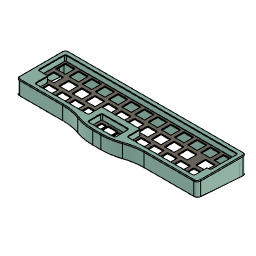
threeu v1 (Autodesk Fusion 360 design; units mm, degrees)
Autodesk Fusion 360 part; units mm, degrees
sketch "plate-2023-07-07T18_42_50.088Z" plane through (0, 0, 0) normal (0, 0, 1) x (1, 0, 0) in component "threeu"
  line L0 (40.625, -3.025) -> (40.625, -16.025)
  line L1 (3.025, -2.525) -> (16.025, -2.525)
  arc A0 (21.575, -16.025) -> (22.075, -16.525) centre (22.075, -16.025) ccw
  arc A1 (59.675, -16.025) -> (60.175, -16.525) centre (60.175, -16.025) ccw
  arc A2 (79.225, -2.525) -> (78.725, -3.025) centre (79.225, -3.025) ccw
  line L2 (98.275, -16.525) -> (111.275, -16.525)
  arc A3 (35.575, -3.025) -> (35.075, -2.525) centre (35.075, -3.025) ccw
  arc A4 (54.125, -16.525) -> (54.625, -16.025) centre (54.125, -16.025) ccw
  line L3 (97.775, -3.025) -> (97.775, -16.025)
  arc A5 (111.775, -3.025) -> (111.275, -2.525) centre (111.275, -3.025) ccw
  arc A6 (111.275, -16.525) -> (111.775, -16.025) centre (111.275, -16.025) ccw
  arc A7 (117.325, -2.525) -> (116.825, -3.025) centre (117.325, -3.025) ccw
  line L4 (136.375, -16.525) -> (149.375, -16.525)
  line L5 (35.575, -3.025) -> (35.575, -16.025)
  line L6 (3.025, -16.525) -> (16.025, -16.525)
  arc A8 (73.175, -16.525) -> (73.675, -16.025) centre (73.175, -16.025) ccw
  line L7 (92.725, -3.025) -> (92.725, -16.025)
  line L8 (135.875, -3.025) -> (135.875, -16.025)
  line L9 (149.875, -3.025) -> (149.875, -16.025)
  line L10 (60.175, -2.525) -> (73.175, -2.525)
  arc A9 (136.375, -2.525) -> (135.875, -3.025) centre (136.375, -3.025) ccw
  line L11 (73.675, -3.025) -> (73.675, -16.025)
  arc A10 (92.225, -16.525) -> (92.725, -16.025) centre (92.225, -16.025) ccw
  arc A11 (16.525, -3.025) -> (16.025, -2.525) centre (16.025, -3.025) ccw
  line L12 (79.225, -2.525) -> (92.225, -2.525)
  line L13 (79.225, -16.525) -> (92.225, -16.525)
  line L14 (22.075, -16.525) -> (35.075, -16.525)
  arc A12 (92.725, -3.025) -> (92.225, -2.525) centre (92.225, -3.025) ccw
  line L15 (111.775, -3.025) -> (111.775, -16.025)
  arc A13 (22.075, -2.525) -> (21.575, -3.025) centre (22.075, -3.025) ccw
  line L16 (21.575, -3.025) -> (21.575, -16.025)
  line L17 (98.275, -2.525) -> (111.275, -2.525)
  arc A14 (73.675, -3.025) -> (73.175, -2.525) centre (73.175, -3.025) ccw
  line L18 (136.375, -2.525) -> (149.375, -2.525)
  arc A15 (3.025, -2.525) -> (2.525, -3.025) centre (3.025, -3.025) ccw
  line L19 (2.525, -3.025) -> (2.525, -16.025)
  line L20 (54.625, -3.025) -> (54.625, -16.025)
  arc A16 (40.625, -16.025) -> (41.125, -16.525) centre (41.125, -16.025) ccw
  line L21 (41.125, -2.525) -> (54.125, -2.525)
  arc A17 (35.075, -16.525) -> (35.575, -16.025) centre (35.075, -16.025) ccw
  arc A18 (16.025, -16.525) -> (16.525, -16.025) centre (16.025, -16.025) ccw
  arc A19 (116.825, -16.025) -> (117.325, -16.525) centre (117.325, -16.025) ccw
  line L22 (174.475, -16.525) -> (187.475, -16.525)
  line L23 (16.525, -3.025) -> (16.525, -16.025)
  arc A20 (60.175, -2.525) -> (59.675, -3.025) centre (60.175, -3.025) ccw
  arc A21 (212.575, -2.525) -> (212.075, -3.025) centre (212.575, -3.025) ccw
  line L24 (130.825, -3.025) -> (130.825, -16.025)
  line L25 (117.325, -2.525) -> (130.325, -2.525)
  line L26 (117.325, -16.525) -> (130.325, -16.525)
  line L27 (22.075, -2.525) -> (35.075, -2.525)
  line L28 (59.675, -3.025) -> (59.675, -16.025)
  arc A22 (149.375, -16.525) -> (149.875, -16.025) centre (149.375, -16.025) ccw
  line L29 (193.025, -3.025) -> (193.025, -16.025)
  arc A23 (245.125, -3.025) -> (244.625, -2.525) centre (244.625, -3.025) ccw
  arc A24 (78.725, -16.025) -> (79.225, -16.525) centre (79.225, -16.025) ccw
  arc A25 (98.275, -2.525) -> (97.775, -3.025) centre (98.275, -3.025) ccw
  arc A26 (41.125, -2.525) -> (40.625, -3.025) centre (41.125, -3.025) ccw
  line L30 (116.825, -3.025) -> (116.825, -16.025)
  arc A27 (231.125, -16.025) -> (231.625, -16.525) centre (231.625, -16.025) ccw
  arc A28 (18.9062, -22.075) -> (18.4062, -21.575) centre (18.4062, -22.075) ccw
  arc A29 (130.825, -3.025) -> (130.325, -2.525) centre (130.325, -3.025) ccw
  arc A30 (130.325, -16.525) -> (130.825, -16.025) centre (130.325, -16.025) ccw
  arc A31 (18.4062, -35.575) -> (18.9062, -35.075) centre (18.4062, -35.075) ccw
  line L31 (45.8875, -21.575) -> (58.8875, -21.575)
  line L32 (154.925, -3.025) -> (154.925, -16.025)
  arc A32 (97.775, -16.025) -> (98.275, -16.525) centre (98.275, -16.025) ccw
  arc A33 (193.525, -2.525) -> (193.025, -3.025) centre (193.525, -3.025) ccw
  arc A34 (40.3375, -22.075) -> (39.8375, -21.575) centre (39.8375, -22.075) ccw
  line L33 (212.075, -3.025) -> (212.075, -16.025)
  line L34 (174.475, -2.525) -> (187.475, -2.525)
  arc A35 (207.025, -3.025) -> (206.525, -2.525) centre (206.525, -3.025) ccw
  line L35 (41.125, -16.525) -> (54.125, -16.525)
  arc A36 (231.625, -2.525) -> (231.125, -3.025) centre (231.625, -3.025) ccw
  arc A37 (54.625, -3.025) -> (54.125, -2.525) centre (54.125, -3.025) ccw
  line L36 (78.725, -3.025) -> (78.725, -16.025)
  line L37 (231.125, -3.025) -> (231.125, -16.025)
  arc A38 (149.875, -3.025) -> (149.375, -2.525) centre (149.375, -3.025) ccw
  arc A39 (135.875, -16.025) -> (136.375, -16.525) centre (136.375, -16.025) ccw
  arc A40 (155.425, -2.525) -> (154.925, -3.025) centre (155.425, -3.025) ccw
  line L38 (26.8375, -21.575) -> (39.8375, -21.575)
  line L39 (26.3375, -22.075) -> (26.3375, -35.075)
  line L40 (18.9063, -22.075) -> (18.9063, -35.075)
  line L41 (60.175, -16.525) -> (73.175, -16.525)
  line L42 (155.425, -16.525) -> (168.425, -16.525)
  arc A41 (2.525, -16.025) -> (3.025, -16.525) centre (3.025, -16.025) ccw
  arc A42 (212.075, -16.025) -> (212.575, -16.525) centre (212.575, -16.025) ccw
  arc A43 (5.4062, -21.575) -> (4.9063, -22.075) centre (5.4062, -22.075) ccw
  line L43 (45.8875, -35.575) -> (58.8875, -35.575)
  line L44 (5.4062, -35.575) -> (18.4063, -35.575)
  line L45 (212.575, -2.525) -> (225.575, -2.525)
  line L46 (59.3875, -22.075) -> (59.3875, -35.075)
  arc A44 (193.025, -16.025) -> (193.525, -16.525) centre (193.525, -16.025) ccw
  line L47 (45.3875, -22.075) -> (45.3875, -35.075)
  line L48 (193.525, -2.525) -> (206.525, -2.525)
  arc A45 (45.8875, -21.575) -> (45.3875, -22.075) centre (45.8875, -22.075) ccw
  line L49 (212.575, -16.525) -> (225.575, -16.525)
  line L50 (187.975, -3.025) -> (187.975, -16.025)
  line L51 (173.975, -3.025) -> (173.975, -16.025)
  arc A46 (187.475, -16.525) -> (187.975, -16.025) centre (187.475, -16.025) ccw
  line L52 (207.025, -3.025) -> (207.025, -16.025)
  arc A47 (168.425, -16.525) -> (168.925, -16.025) centre (168.425, -16.025) ccw
  line L53 (245.125, -3.025) -> (245.125, -16.025)
  line L54 (226.075, -3.025) -> (226.075, -16.025)
  arc A48 (225.575, -16.525) -> (226.075, -16.025) centre (225.575, -16.025) ccw
  line L55 (26.8375, -35.575) -> (39.8375, -35.575)
  line L56 (168.925, -3.025) -> (168.925, -16.025)
  line L57 (231.625, -2.525) -> (244.625, -2.525)
  line L58 (4.9062, -22.075) -> (4.9062, -35.075)
  line L59 (193.525, -16.525) -> (206.525, -16.525)
  arc A49 (174.475, -2.525) -> (173.975, -3.025) centre (174.475, -3.025) ccw
  arc A50 (226.075, -3.025) -> (225.575, -2.525) centre (225.575, -3.025) ccw
  arc A51 (4.9062, -35.075) -> (5.4062, -35.575) centre (5.4062, -35.075) ccw
  line L60 (40.3375, -22.075) -> (40.3375, -35.075)
  line L61 (5.4062, -21.575) -> (18.4063, -21.575)
  arc A52 (168.925, -3.025) -> (168.425, -2.525) centre (168.425, -3.025) ccw
  line L62 (231.625, -16.525) -> (244.625, -16.525)
  line L63 (155.425, -2.525) -> (168.425, -2.525)
  arc A53 (26.3375, -35.075) -> (26.8375, -35.575) centre (26.8375, -35.075) ccw
  arc A54 (39.8375, -35.575) -> (40.3375, -35.075) centre (39.8375, -35.075) ccw
  arc A55 (187.975, -3.025) -> (187.475, -2.525) centre (187.475, -3.025) ccw
  arc A56 (244.625, -16.525) -> (245.125, -16.025) centre (244.625, -16.025) ccw
  arc A57 (26.8375, -21.575) -> (26.3375, -22.075) centre (26.8375, -22.075) ccw
  arc A58 (160.1875, -21.575) -> (159.6875, -22.075) centre (160.1875, -22.075) ccw
  arc A59 (173.975, -16.025) -> (174.475, -16.525) centre (174.475, -16.025) ccw
  arc A60 (206.525, -16.525) -> (207.025, -16.025) centre (206.525, -16.025) ccw
  line L64 (103.0375, -21.575) -> (116.0375, -21.575)
  line L65 (192.7375, -22.075) -> (192.7375, -35.075)
  line L66 (160.1875, -21.575) -> (173.1875, -21.575)
  arc A61 (178.7375, -35.075) -> (179.2375, -35.575) centre (179.2375, -35.075) ccw
  arc A62 (154.925, -16.025) -> (155.425, -16.525) centre (155.425, -16.025) ccw
  arc A63 (140.6375, -35.075) -> (141.1375, -35.575) centre (141.1375, -35.075) ccw
  arc A64 (135.5875, -22.075) -> (135.0875, -21.575) centre (135.0875, -22.075) ccw
  arc A65 (141.1375, -21.575) -> (140.6375, -22.075) centre (141.1375, -22.075) ccw
  line L67 (141.1375, -21.575) -> (154.1375, -21.575)
  arc A66 (192.2375, -35.575) -> (192.7375, -35.075) centre (192.2375, -35.075) ccw
  line L68 (64.9375, -35.575) -> (77.9375, -35.575)
  arc A67 (159.6875, -35.075) -> (160.1875, -35.575) centre (160.1875, -35.075) ccw
  line L69 (159.6875, -22.075) -> (159.6875, -35.075)
  line L70 (83.9875, -35.575) -> (96.9875, -35.575)
  line L71 (64.9375, -21.575) -> (77.9375, -21.575)
  arc A68 (192.7375, -22.075) -> (192.2375, -21.575) centre (192.2375, -22.075) ccw
  line L72 (198.2875, -21.575) -> (211.2875, -21.575)
  line L73 (97.4875, -22.075) -> (97.4875, -35.075)
  arc A69 (59.3875, -22.075) -> (58.8875, -21.575) centre (58.8875, -22.075) ccw
  arc A70 (58.8875, -35.575) -> (59.3875, -35.075) centre (58.8875, -35.075) ccw
  line L74 (179.2375, -35.575) -> (192.2375, -35.575)
  arc A71 (154.6375, -22.075) -> (154.1375, -21.575) centre (154.1375, -22.075) ccw
  line L75 (179.2375, -21.575) -> (192.2375, -21.575)
  line L76 (197.7875, -22.075) -> (197.7875, -35.075)
  line L77 (140.6375, -22.075) -> (140.6375, -35.075)
  line L78 (198.2875, -35.575) -> (211.2875, -35.575)
  line L79 (135.5875, -22.075) -> (135.5875, -35.075)
  line L80 (102.5375, -22.075) -> (102.5375, -35.075)
  arc A72 (173.6875, -22.075) -> (173.1875, -21.575) centre (173.1875, -22.075) ccw
  line L81 (154.6375, -22.075) -> (154.6375, -35.075)
  arc A73 (64.9375, -21.575) -> (64.4375, -22.075) centre (64.9375, -22.075) ccw
  line L82 (160.1875, -35.575) -> (173.1875, -35.575)
  arc A74 (179.2375, -21.575) -> (178.7375, -22.075) centre (179.2375, -22.075) ccw
  line L83 (211.7875, -22.075) -> (211.7875, -35.075)
  arc A75 (122.0875, -21.575) -> (121.5875, -22.075) centre (122.0875, -22.075) ccw
  arc A76 (97.4875, -22.075) -> (96.9875, -21.575) centre (96.9875, -22.075) ccw
  line L84 (122.0875, -35.575) -> (135.0875, -35.575)
  line L85 (178.7375, -22.075) -> (178.7375, -35.075)
  arc A77 (103.0375, -21.575) -> (102.5375, -22.075) centre (103.0375, -22.075) ccw
  line L86 (83.9875, -21.575) -> (96.9875, -21.575)
  line L87 (116.5375, -22.075) -> (116.5375, -35.075)
  line L88 (83.4875, -22.075) -> (83.4875, -35.075)
  line L89 (141.1375, -35.575) -> (154.1375, -35.575)
  arc A78 (96.9875, -35.575) -> (97.4875, -35.075) centre (96.9875, -35.075) ccw
  line L90 (17.3125, -40.625) -> (30.3125, -40.625)
  arc A79 (223.9813, -35.075) -> (224.4813, -35.575) centre (224.4813, -35.075) ccw
  line L91 (103.0375, -35.575) -> (116.0375, -35.575)
  arc A80 (116.5375, -22.075) -> (116.0375, -21.575) centre (116.0375, -22.075) ccw
  arc A81 (77.9375, -35.575) -> (78.4375, -35.075) centre (77.9375, -35.075) ccw
  line L92 (122.0875, -21.575) -> (135.0875, -21.575)
  arc A82 (78.4375, -22.075) -> (77.9375, -21.575) centre (77.9375, -22.075) ccw
  arc A83 (188.7625, -40.625) -> (188.2625, -41.125) centre (188.7625, -41.125) ccw
  arc A84 (45.3875, -35.075) -> (45.8875, -35.575) centre (45.8875, -35.075) ccw
  arc A85 (121.5875, -35.075) -> (122.0875, -35.575) centre (122.0875, -35.075) ccw
  line L93 (183.2125, -41.125) -> (183.2125, -54.125)
  arc A86 (154.1375, -35.575) -> (154.6375, -35.075) centre (154.1375, -35.075) ccw
  line L94 (173.6875, -22.075) -> (173.6875, -35.075)
  arc A87 (87.9625, -41.125) -> (87.4625, -40.625) centre (87.4625, -41.125) ccw
  arc A88 (198.2875, -21.575) -> (197.7875, -22.075) centre (198.2875, -22.075) ccw
  line L95 (121.5875, -22.075) -> (121.5875, -35.075)
  arc A89 (83.4875, -35.075) -> (83.9875, -35.575) centre (83.9875, -35.075) ccw
  arc A90 (68.9125, -41.125) -> (68.4125, -40.625) centre (68.4125, -41.125) ccw
  arc A91 (211.7875, -22.075) -> (211.2875, -21.575) centre (211.2875, -22.075) ccw
  arc A92 (164.1625, -41.125) -> (163.6625, -40.625) centre (163.6625, -41.125) ccw
  line L96 (150.6625, -40.625) -> (163.6625, -40.625)
  arc A93 (237.9813, -22.075) -> (237.4813, -21.575) centre (237.4813, -22.075) ccw
  line L97 (78.4375, -22.075) -> (78.4375, -35.075)
  line L98 (64.4375, -22.075) -> (64.4375, -35.075)
  line L99 (202.2625, -41.125) -> (202.2625, -54.125)
  arc A94 (83.9875, -21.575) -> (83.4875, -22.075) centre (83.9875, -22.075) ccw
  arc A95 (173.1875, -35.575) -> (173.6875, -35.075) centre (173.1875, -35.075) ccw
  arc A96 (116.0375, -35.575) -> (116.5375, -35.075) centre (116.0375, -35.075) ccw
  arc A97 (135.0875, -35.575) -> (135.5875, -35.075) centre (135.0875, -35.075) ccw
  arc A98 (87.4625, -54.625) -> (87.9625, -54.125) centre (87.4625, -54.125) ccw
  arc A99 (64.4375, -35.075) -> (64.9375, -35.575) centre (64.9375, -35.075) ccw
  arc A100 (102.5375, -35.075) -> (103.0375, -35.575) centre (103.0375, -35.075) ccw
  line L100 (49.8625, -41.125) -> (49.8625, -54.125)
  arc A101 (16.8125, -54.125) -> (17.3125, -54.625) centre (17.3125, -54.125) ccw
  line L101 (36.3625, -40.625) -> (49.3625, -40.625)
  arc A102 (49.3625, -54.625) -> (49.8625, -54.125) centre (49.3625, -54.125) ccw
  line L102 (74.4625, -54.625) -> (87.4625, -54.625)
  line L103 (223.9812, -22.075) -> (223.9812, -35.075)
  line L104 (16.8125, -41.125) -> (16.8125, -54.125)
  arc A103 (17.3125, -40.625) -> (16.8125, -41.125) centre (17.3125, -41.125) ccw
  arc A104 (224.4813, -21.575) -> (223.9813, -22.075) centre (224.4813, -22.075) ccw
  arc A105 (36.3625, -40.625) -> (35.8625, -41.125) centre (36.3625, -41.125) ccw
  line L105 (54.9125, -41.125) -> (54.9125, -54.125)
  arc A106 (55.4125, -40.625) -> (54.9125, -41.125) centre (55.4125, -41.125) ccw
  line L106 (30.8125, -41.125) -> (30.8125, -54.125)
  arc A107 (73.9625, -54.125) -> (74.4625, -54.625) centre (74.4625, -54.125) ccw
  arc A108 (68.4125, -54.625) -> (68.9125, -54.125) centre (68.4125, -54.125) ccw
  line L107 (55.4125, -40.625) -> (68.4125, -40.625)
  arc A109 (197.7875, -35.075) -> (198.2875, -35.575) centre (198.2875, -35.075) ccw
  line L108 (36.3625, -54.625) -> (49.3625, -54.625)
  line L109 (164.1625, -41.125) -> (164.1625, -54.125)
  arc A110 (150.6625, -40.625) -> (150.1625, -41.125) centre (150.6625, -41.125) ccw
  arc A111 (30.8125, -41.125) -> (30.3125, -40.625) centre (30.3125, -41.125) ccw
  line L110 (237.9813, -22.075) -> (237.9812, -35.075)
  arc A112 (237.4813, -35.575) -> (237.9813, -35.075) centre (237.4813, -35.075) ccw
  line L111 (35.8625, -41.125) -> (35.8625, -54.125)
  line L112 (150.6625, -54.625) -> (163.6625, -54.625)
  line L113 (74.4625, -40.625) -> (87.4625, -40.625)
  line L114 (55.4125, -54.625) -> (68.4125, -54.625)
  line L115 (169.7125, -40.625) -> (182.7125, -40.625)
  arc A113 (169.7125, -40.625) -> (169.2125, -41.125) centre (169.7125, -41.125) ccw
  arc A114 (169.2125, -54.125) -> (169.7125, -54.625) centre (169.7125, -54.125) ccw
  arc A115 (182.7125, -54.625) -> (183.2125, -54.125) centre (182.7125, -54.125) ccw
  arc A116 (211.2875, -35.575) -> (211.7875, -35.075) centre (211.2875, -35.075) ccw
  arc A117 (30.3125, -54.625) -> (30.8125, -54.125) centre (30.3125, -54.125) ccw
  line L116 (68.9125, -41.125) -> (68.9125, -54.125)
  line L117 (73.9625, -41.125) -> (73.9625, -54.125)
  arc A118 (150.1625, -54.125) -> (150.6625, -54.625) centre (150.6625, -54.125) ccw
  line L118 (150.1625, -41.125) -> (150.1625, -54.125)
  line L119 (169.2125, -41.125) -> (169.2125, -54.125)
  arc A119 (183.2125, -41.125) -> (182.7125, -40.625) centre (182.7125, -41.125) ccw
  line L120 (224.4813, -35.575) -> (237.4813, -35.575)
  line L121 (87.9625, -41.125) -> (87.9625, -54.125)
  line L122 (17.3125, -54.625) -> (30.3125, -54.625)
  arc A120 (54.9125, -54.125) -> (55.4125, -54.625) centre (55.4125, -54.125) ccw
  arc A121 (163.6625, -54.625) -> (164.1625, -54.125) centre (163.6625, -54.125) ccw
  arc A122 (35.8625, -54.125) -> (36.3625, -54.625) centre (36.3625, -54.125) ccw
  arc A123 (49.8625, -41.125) -> (49.3625, -40.625) centre (49.3625, -41.125) ccw
  line L123 (188.2625, -41.125) -> (188.2625, -54.125)
  arc A124 (74.4625, -40.625) -> (73.9625, -41.125) centre (74.4625, -41.125) ccw
  line L124 (224.4813, -21.575) -> (237.4813, -21.575)
  line L125 (169.7125, -54.625) -> (182.7125, -54.625)
  line L126 (188.7625, -40.625) -> (201.7625, -40.625)
  line L127 (188.7625, -54.625) -> (201.7625, -54.625)
  line L128 (112.0625, -50.65) -> (112.0625, -63.65)
  line L129 (128.0005, -51.15) -> (134.0005, -51.15)
  arc A125 (110.6245, -51.65) -> (110.1245, -51.15) centre (110.1245, -51.65) ccw
  arc A126 (134.5005, -51.65) -> (134.0005, -51.15) centre (134.0005, -51.65) ccw
  arc A127 (221.3125, -41.125) -> (220.8125, -40.625) centre (220.8125, -41.125) ccw
  line L130 (100.0125, -66.675) -> (138.1125, -66.675)
  arc A128 (112.0625, -63.65) -> (112.5625, -64.15) centre (112.5625, -63.65) ccw
  arc A129 (201.7625, -54.625) -> (202.2625, -54.125) centre (201.7625, -54.125) ccw
  line L131 (134.5005, -51.65) -> (134.5005, -65.65)
  arc A130 (239.8625, -54.625) -> (240.3625, -54.125) centre (239.8625, -54.125) ccw
  line L132 (127.5005, -51.65) -> (127.5005, -65.65)
  line L133 (0, 0) -> (247.65, 0)
  arc A131 (127.5005, -65.65) -> (128.0005, -66.15) centre (128.0005, -65.65) ccw
  line L134 (126.0625, -50.65) -> (126.0625, -63.65)
  line L135 (226.8625, -40.625) -> (239.8625, -40.625)
  arc A132 (226.8625, -40.625) -> (226.3625, -41.125) centre (226.8625, -41.125) ccw
  arc A133 (110.1245, -66.15) -> (110.6245, -65.65) centre (110.1245, -65.65) ccw
  line L136 (240.3625, -41.125) -> (240.3625, -54.125)
  arc A134 (226.3625, -54.125) -> (226.8625, -54.625) centre (226.8625, -54.125) ccw
  line L137 (221.3125, -41.125) -> (221.3125, -54.125)
  arc A135 (125.5625, -64.15) -> (126.0625, -63.65) centre (125.5625, -63.65) ccw
  line L138 (128.0005, -66.15) -> (134.0005, -66.15)
  arc A136 (220.8125, -54.625) -> (221.3125, -54.125) centre (220.8125, -54.125) ccw
  arc A137 (126.0625, -50.65) -> (125.5625, -50.15) centre (125.5625, -50.65) ccw
  line L139 (104.1245, -66.15) -> (110.1245, -66.15)
  arc A138 (112.5625, -50.15) -> (112.0625, -50.65) centre (112.5625, -50.65) ccw
  line L140 (110.6245, -51.65) -> (110.6245, -65.65)
  arc A139 (103.6245, -65.65) -> (104.1245, -66.15) centre (104.1245, -65.65) ccw
  arc A140 (202.2625, -41.125) -> (201.7625, -40.625) centre (201.7625, -41.125) ccw
  line L141 (226.8625, -54.625) -> (239.8625, -54.625)
  line L142 (207.8125, -54.625) -> (220.8125, -54.625)
  arc A141 (207.8125, -40.625) -> (207.3125, -41.125) centre (207.8125, -41.125) ccw
  line L143 (226.3625, -41.125) -> (226.3625, -54.125)
  arc A142 (207.3125, -54.125) -> (207.8125, -54.625) centre (207.8125, -54.125) ccw
  arc A143 (188.2625, -54.125) -> (188.7625, -54.625) centre (188.7625, -54.125) ccw
  line L144 (207.8125, -40.625) -> (220.8125, -40.625)
  line L145 (112.5625, -50.15) -> (125.5625, -50.15)
  line L146 (104.1245, -51.15) -> (110.1245, -51.15)
  arc A144 (134.0005, -66.15) -> (134.5005, -65.65) centre (134.0005, -65.65) ccw
  line L147 (0, -38.1) -> (0, 0)
  arc A145 (128.0005, -51.15) -> (127.5005, -51.65) centre (128.0005, -51.65) ccw
  line L148 (207.3125, -41.125) -> (207.3125, -54.125)
  line L149 (103.6245, -51.65) -> (103.6245, -65.65)
  arc A146 (104.1245, -51.15) -> (103.6245, -51.65) centre (104.1245, -51.65) ccw
  arc A147 (240.3625, -41.125) -> (239.8625, -40.625) centre (239.8625, -41.125) ccw
  line L150 (112.5625, -64.15) -> (125.5625, -64.15)
  line L151 (247.65, -38.1) -> (247.65, 0)
  line L152 (33.3375, -57.15) -> (14.2875, -57.15)
  line L153 (14.2875, -57.15) -> (14.2875, -38.1)
  line L154 (14.2875, -38.1) -> (33.3375, -57.15) construction
  line L155 (33.3375, -38.1) -> (14.2875, -57.15) construction
  line L156 (242.8875, -57.15) -> (223.8375, -57.15)
  line L157 (242.8875, -38.1) -> (242.8875, -57.15)
  line L158 (242.8875, -57.15) -> (223.8375, -38.1) construction
  line L159 (223.8375, -57.15) -> (242.8875, -38.1) construction
  line L160 (242.8875, -38.1) -> (247.65, -38.1)
  line L161 (138.1125, -66.675) -> (100.0125, -66.675)
  line L162 (100.0125, -66.675) -> (100.0125, -47.625)
  line L163 (100.0125, -47.625) -> (138.1125, -47.625)
  line L164 (138.1125, -47.625) -> (138.1125, -66.675)
  line L165 (138.1125, -66.675) -> (100.0125, -47.625) construction
  line L166 (100.0125, -66.675) -> (138.1125, -47.625) construction
  line L167 (90.4875, -57.15) -> (71.4375, -57.15)
  line L168 (90.4875, -38.1) -> (90.4875, -57.15)
  line L169 (90.4875, -57.15) -> (71.4375, -38.1) construction
  line L170 (71.4375, -57.15) -> (90.4875, -38.1) construction
  line L171 (147.6375, -57.15) -> (166.6875, -57.15)
  line L172 (147.6375, -38.1) -> (147.6375, -57.15)
  line L173 (147.6375, -57.15) -> (166.6875, -38.1) construction
  line L174 (166.6875, -57.15) -> (147.6375, -38.1) construction
  line L175 (147.6375, -38.1) -> (90.4875, -38.1)
  line L176 (71.4375, -57.15) -> (33.3375, -57.15)
  line L177 (14.2875, -38.1) -> (0, -38.1)
  line L178 (166.6875, -57.15) -> (223.8375, -57.15)
  line L179 (138.1125, -66.675) -> (147.6375, -57.15)
  line L180 (100.0125, -66.675) -> (90.4875, -57.15)
  line L181 (141.012, -73.675) -> (150.537, -64.15)
  line L182 (150.537, -64.15) -> (166.6875, -64.15)
  line L183 (166.6875, -64.15) -> (223.8375, -64.15)
  line L184 (249.8875, -64.15) -> (223.8375, -64.15)
  line L185 (254.65, -45.1) -> (254.65, 7)
  line L186 (-7, 7) -> (254.65, 7)
  line L187 (-7, -45.1) -> (-7, 7)
  line L188 (33.3375, -64.15) -> (7.2875, -64.15)
  line L189 (71.4375, -64.15) -> (33.3375, -64.15)
  line L190 (87.588, -64.15) -> (71.4375, -64.15)
  line L191 (97.113, -73.675) -> (87.588, -64.15)
  line L192 (97.113, -73.675) -> (141.012, -73.675)
  line L193 (7.2875, -64.15) -> (-7, -64.15)
  line L194 (-7, -64.15) -> (-7, -45.1)
  line L195 (249.8875, -64.15) -> (254.65, -64.15)
  line L196 (254.65, -64.15) -> (254.65, -45.1)
  line L197 (138.5267, -67.675) -> (148.0517, -58.15)
  line L198 (148.0517, -58.15) -> (166.6875, -58.15)
  line L199 (166.6875, -58.15) -> (223.8375, -58.15)
  line L200 (243.8875, -58.15) -> (223.8375, -58.15)
  line L201 (243.8875, -39.1) -> (243.8875, -58.15)
  line L202 (243.8875, -39.1) -> (248.65, -39.1)
  line L203 (248.65, -39.1) -> (248.65, 1)
  line L204 (-1, 1) -> (248.65, 1)
  line L205 (-1, -39.1) -> (-1, 1)
  line L206 (13.2875, -39.1) -> (-1, -39.1)
  line L207 (13.2875, -58.15) -> (13.2875, -39.1)
  line L208 (33.3375, -58.15) -> (13.2875, -58.15)
  line L209 (71.4375, -58.15) -> (33.3375, -58.15)
  line L210 (90.0733, -58.15) -> (71.4375, -58.15)
  line L211 (99.5983, -67.675) -> (90.0733, -58.15)
  line L212 (99.5983, -67.675) -> (138.5267, -67.675)
  line L213 (242.8875, -57.15) -> (247.65, -57.15)
  line L214 (247.65, -57.15) -> (247.65, -38.1)
  line L215 (14.2875, -57.15) -> (0, -57.15)
  line L216 (0, -57.15) -> (0, -38.1)
  line L217 (247.65, 0) -> (252.65, 0)
  line L218 (252.65, -4) -> (247.65, -4)
  line L219 (247.65, -4) -> (247.65, 0)
  line L220 (252.65, -0.75) -> (250.15, -0.75)
  line L221 (250.15, -3.25) -> (252.65, -3.25)
  line L222 (252.65, 0) -> (252.65, -0.75)
  line L223 (252.65, -3.25) -> (252.65, -4)
  arc A148 (250.15, -0.75) -> (250.15, -3.25) centre (250.15, -2) ccw
  line L224 (254.65, 7) -> (254.65, -64.15) construction
  line L225 (254.65, -28.575) -> (248.65, -28.575) construction
  line L226 (248.65, 4.2629) -> (-1, 4.2629) construction
  line L227 (123.825, 4.2629) -> (123.825, 7) construction
  line L228 (-5, -3.25) -> (-5, -4)
  line L229 (0, -4) -> (0, 0)
  line L230 (-5, -4) -> (0, -4)
  line L231 (-5, 0) -> (-5, -0.75)
  line L232 (0, 0) -> (-5, 0)
  arc A149 (-2.5, -3.25) -> (-2.5, -0.75) centre (-2.5, -2) ccw
  line L233 (-5, -0.75) -> (-2.5, -0.75)
  line L234 (-2.5, -3.25) -> (-5, -3.25)
  line L235 (247.65, -57.15) -> (252.65, -57.15)
  arc A150 (250.15, -53.9) -> (250.15, -56.4) centre (250.15, -55.15) ccw
  line L236 (252.65, -53.15) -> (247.65, -53.15)
  line L237 (252.65, -57.15) -> (252.65, -56.4)
  line L238 (250.15, -53.9) -> (252.65, -53.9)
  line L239 (247.65, -53.15) -> (247.65, -57.15)
  line L240 (252.65, -56.4) -> (250.15, -56.4)
  line L241 (252.65, -53.9) -> (252.65, -53.15)
  line L242 (-2.5, -53.9) -> (-5, -53.9)
  line L243 (-5, -53.15) -> (0, -53.15)
  line L244 (-5, -56.4) -> (-2.5, -56.4)
  line L245 (-5, -53.9) -> (-5, -53.15)
  line L246 (-5, -57.15) -> (-5, -56.4)
  arc A151 (-2.5, -56.4) -> (-2.5, -53.9) centre (-2.5, -55.15) ccw
  line L247 (0, -53.15) -> (0, -57.15)
  line L248 (0, -57.15) -> (-5, -57.15)
  line L249 (-1, -39.1) -> (13.2875, -39.1)
  line L250 (13.2875, -39.1) -> (13.2875, -58.15)
  line L251 (13.2875, -58.15) -> (-1, -58.15)
  line L252 (-1, -58.15) -> (-1, -39.1)
  line L253 (248.65, -39.1) -> (243.8875, -39.1)
  line L254 (243.8875, -39.1) -> (243.8875, -58.15)
  line L255 (243.8875, -58.15) -> (248.65, -58.15)
  line L256 (248.65, -58.15) -> (248.65, -39.1)
  point P0 (23.8125, -47.625)
  point P1 (233.3625, -47.625)
  point P2 (119.0625, -57.15)
  point P3 (80.9625, -47.625)
  point P4 (157.1625, -47.625)
  point P5 (252.65, -2)
  point P6 (-5, -2)
  point P7 (252.65, -55.15)
  point P8 (0, -57.15)
  point P9 (-5, -55.15)
  dimension "d1" = 19.05
  dimension "d2" = 19.05
  dimension "d3" = 19.05
  dimension "d4" = 19.05
  dimension "d5" = 38.1
  dimension "d6" = 19.05
  dimension "d7" = 19.05
  dimension "d8" = 19.05
  dimension "d10" = 1
  dimension "d13" = 5
  dimension "d14" = 4
  constraint coincident L154 P0
  constraint coincident L155 P0
  constraint horizontal L156
  constraint coincident L158 P1
  constraint coincident L159 P1
  constraint perpendicular L151 L160
  constraint horizontal L161
  constraint perpendicular L161 L162
  constraint parallel L161 L163
  constraint parallel L162 L164
  constraint coincident L165 P2
  constraint coincident L166 P2
  constraint horizontal L167
  constraint coincident L169 P3
  constraint coincident L170 P3
  constraint horizontal L171
  constraint coincident L173 P4
  constraint coincident L174 P4
  constraint perpendicular L168 L175
  constraint perpendicular L147 L177
  constraint parallel L173 L179
  constraint perpendicular L179 L180
  constraint horizontal L193
  constraint vertical L194
  constraint horizontal L195
  constraint vertical L196
  constraint horizontal L213
  constraint vertical L214
  constraint horizontal L215
  constraint vertical L216
  constraint horizontal L217
  constraint vertical L222
  constraint horizontal L218
  constraint vertical L219
  constraint horizontal L221
  constraint coincident L221.end L222
  constraint collinear L222 L223
  constraint coincident P5 L222
  constraint tangent L221 A148
  constraint perpendicular L195 L224
  constraint midpoint L224 L225.start
  constraint coincident L203 L225.end
  constraint perpendicular L203 L225
  constraint perpendicular L205 L226
  constraint midpoint L226 L227.start
  constraint midpoint L186 L227.end
  constraint perpendicular L186 L227
  constraint symmetric L133.end L227 L133.start
  constraint symmetric L217.end L227 L231.start
  constraint symmetric L218.start L227 L228.end
  constraint symmetric L218.end L227 L229.start
  constraint symmetric L221.start L227 A149.start
  constraint symmetric L220.end L227 A149.end
  constraint symmetric P5 L227 P6
  constraint symmetric L220.start L227 L231.end
  constraint symmetric L221.end L227 L228.start
  constraint symmetric A148 L227 A149
  constraint symmetric L133.start L225 P8
  constraint symmetric L133.end L225 L213.end
  constraint symmetric L217.end L225 L235.end
  constraint symmetric L218.start L225 L236.start
  constraint symmetric L218.end L225 L236.end
  constraint symmetric L221.start L225 A150.start
  constraint symmetric L220.end L225 A150.end
  constraint symmetric P5 L225 P7
  constraint symmetric L220.start L225 L237.end
  constraint symmetric L221.end L225 L238.end
  constraint symmetric A148 L225 A150
  constraint symmetric L225 L231.start L246.start
  constraint symmetric L225 L133.start P8
  constraint symmetric L225 L229.start L243.end
  constraint symmetric L225 L228.end L243.start
  constraint symmetric L225 P6 P9
  constraint symmetric L225 A149.start L242.start
  constraint symmetric L225 A149.end L244.end
  constraint symmetric L225 L231.end L244.start
  constraint symmetric L225 L228.start L242.end
  constraint symmetric L225 A149 A151
  constraint horizontal L249
  constraint vertical L250
  constraint horizontal L251
  constraint vertical L252
  constraint horizontal L253
  constraint vertical L254
  constraint horizontal L255
  constraint vertical L256
  measures "d1" distance of L152.start L152.end
  measures "d2" distance of L155.start L152.start
  measures "d3" distance of L158.end L157.start
  measures "d4" distance of L156.end L158.end
  measures "d5" distance of L162.end L163.end
  measures "d6" distance of L169.end L168.start
  measures "d7" distance of L167.end L169.end
  measures "d8" distance of L173.end L172.start
  measures "d13" distance of L133.end L217.end
  measures "d14" distance of L133.end L218.end
extrude "Extrude1" add sketch "plate-2023-07-07T18_42_50.088Z" along normal blind 7.8 contours L162 L163 L164 L168 L172 L175 L179 L180 | L130 L152 L156 L161 L167 L171 L176 L178 L179 L180 L197 L198 L199 L200 L201 L207 L208 L209 L210 L211 L212 L213 L215 L250 L254 | L153 L177 L206 L207 L215 L216 L249 L250 | L157 L160 L201 L202 L213 L214 L253 L254 | L206 L207 L215 L216 L247 L249 L250 | L207 L215 L248 L250 L251 L252 | L201 L213 L235 L254 L255 L256 | L201 L202 L213 L214 L239 L253 L254 | L147 L205 L206 L216 L230 L249 | L216 L243 L247 L248 L252 | L151 L202 L203 L214 L218 L253 | L214 L235 L236 L239 L256 | L147 L205 L229 L230 L232 | L206 L216 L243 L249 L252 | L242 L243 L244 L245 L246 A151 L248 L252 | L151 L203 L217 L218 L219 | L202 L214 L236 L253 L256 | L235 A150 L236 L237 L238 L240 L241 L256 | L133 L203 L204 L205 L217 L232 | L205 L228 L230 L231 L232 A149 L233 L234 | L203 L217 L218 L220 L221 L222 L223 A148 | L181 L182 L183 L184 L185 L186 L187 L188 L189 L190 L191 L192 L193 L194 L195 L196 makes body 1 in component "threeu"
extrude "Extrude2" add sketch "plate-2023-07-07T18_42_50.088Z" against normal blind 12 separate body contours L181 L182 L183 L184 L185 L186 L187 L188 L189 L190 L191 L192 L193 L194 L195 L196 makes body 2 in component "threeu"
sketch "Sketch2" plane through (0, 0, -12) normal (0, 0, -1) x (1, 0, 0) in component "threeu"
  line L0 (148.0517, 58.15) -> (248.65, 58.15)
  line L1 (248.65, 58.15) -> (248.65, 57.15)
  line L2 (248.65, 57.15) -> (252.65, 57.15)
  line L3 (252.65, 57.15) -> (252.65, 56.4)
  line L4 (252.65, 56.4) -> (250.15, 56.4)
  arc A0 (250.15, 56.4) -> (250.15, 53.9) centre (250.15, 55.15) ccw
  line L5 (250.15, 53.9) -> (252.65, 53.9)
  line L6 (252.65, 53.9) -> (252.65, 53.15)
  line L7 (252.65, 53.15) -> (248.65, 53.15)
  line L8 (248.65, 53.15) -> (248.65, 4)
  line L9 (248.65, 4) -> (252.65, 4)
  line L10 (252.65, 4) -> (252.65, 3.25)
  line L11 (252.65, 3.25) -> (250.15, 3.25)
  arc A1 (250.15, 3.25) -> (250.15, 0.75) centre (250.15, 2) ccw
  line L12 (250.15, 0.75) -> (252.65, 0.75)
  line L13 (252.65, 0.75) -> (252.65, 0)
  line L14 (252.65, 0) -> (248.65, 0)
  line L15 (248.65, 0) -> (248.65, -1)
  line L16 (248.65, -1) -> (-1, -1)
  line L17 (-1, -1) -> (-1, 0)
  line L18 (-1, 0) -> (-5, 0)
  line L19 (-5, 0) -> (-5, 0.75)
  line L20 (-5, 0.75) -> (-2.5, 0.75)
  arc A2 (-2.5, 0.75) -> (-2.5, 3.25) centre (-2.5, 2) ccw
  line L21 (-2.5, 3.25) -> (-5, 3.25)
  line L22 (-5, 3.25) -> (-5, 4)
  line L23 (-5, 4) -> (-1, 4)
  line L24 (-1, 4) -> (-1, 53.15)
  line L25 (-1, 53.15) -> (-5, 53.15)
  line L26 (-5, 53.15) -> (-5, 53.9)
  line L27 (-5, 53.9) -> (-2.5, 53.9)
  arc A3 (-2.5, 53.9) -> (-2.5, 56.4) centre (-2.5, 55.15) ccw
  line L28 (-2.5, 56.4) -> (-5, 56.4)
  line L29 (-5, 56.4) -> (-5, 57.15)
  line L30 (-5, 57.15) -> (-1, 57.15)
  line L31 (-1, 57.15) -> (-1, 58.15)
  line L32 (-1, 58.15) -> (90.0733, 58.15)
  line L33 (90.0733, 58.15) -> (99.5983, 67.675)
  line L34 (99.5983, 67.675) -> (138.5267, 67.675)
  line L35 (138.5267, 67.675) -> (148.0517, 58.15)
  line L36 (254.65, 64.15) -> (150.537, 64.15)
  line L37 (150.537, 64.15) -> (141.012, 73.675)
  line L38 (141.012, 73.675) -> (97.113, 73.675)
  line L39 (97.113, 73.675) -> (87.588, 64.15)
  line L40 (87.588, 64.15) -> (-7, 64.15)
  line L41 (-7, 64.15) -> (-7, -7)
  line L42 (-7, -7) -> (254.65, -7)
  line L43 (254.65, -7) -> (254.65, 64.15)
  line L44 (-5, 0) -> (252.65, 0)
  line L45 (252.65, 0) -> (252.65, 57.15)
  line L46 (252.65, 57.15) -> (-5, 57.15)
  line L47 (-5, 57.15) -> (-5, 0)
  constraint horizontal L44
  constraint vertical L45
  constraint horizontal L46
  constraint vertical L47
  constraint coincident L2.end L3.start
  constraint coincident L18.end L19.start
extrude "Extrude3" cut sketch "Sketch2" against normal blind 12 contours L4 A0 L5 L45 | L27 A3 L28 L47 | L11 A1 L12 L45 | L20 A2 L21 L47 bodies 2 in component "threeu"
sketch "Sketch3" plane through (0, 0, -12) normal (0, 0, -1) x (1, 0, 0) in component "threeu"
  line L0 (252.65, 57.15) -> (252.65, 53.15)
  line L1 (252.65, 53.15) -> (248.65, 53.15)
  line L2 (248.65, 53.15) -> (248.65, 4)
  line L3 (248.65, 4) -> (252.65, 4)
  line L4 (252.65, 4) -> (252.65, 0)
  line L5 (252.65, 0) -> (248.65, 0)
  line L6 (248.65, 0) -> (248.65, -1)
  line L7 (248.65, -1) -> (-1, -1)
  line L8 (-1, -1) -> (-1, 0)
  line L9 (-1, 0) -> (-5, 0)
  line L10 (-5, 0) -> (-5, 4)
  line L11 (-5, 4) -> (-1, 4)
  line L12 (-1, 4) -> (-1, 53.15)
  line L13 (-1, 53.15) -> (-5, 53.15)
  line L14 (-5, 53.15) -> (-5, 57.15)
  line L15 (-5, 57.15) -> (-1, 57.15)
  line L16 (-1, 57.15) -> (-1, 58.15)
  line L17 (-1, 58.15) -> (90.0733, 58.15)
  line L18 (90.0733, 58.15) -> (99.5983, 67.675)
  line L19 (99.5983, 67.675) -> (138.5267, 67.675)
  line L20 (138.5267, 67.675) -> (148.0517, 58.15)
  line L21 (148.0517, 58.15) -> (248.65, 58.15)
  line L22 (248.65, 58.15) -> (248.65, 57.15)
  line L23 (248.65, 57.15) -> (252.65, 57.15)
  line L24 (254.65, 64.15) -> (150.537, 64.15)
  line L25 (150.537, 64.15) -> (141.012, 73.675)
  line L26 (141.012, 73.675) -> (97.113, 73.675)
  line L27 (97.113, 73.675) -> (87.588, 64.15)
  line L28 (87.588, 64.15) -> (-7, 64.15)
  line L29 (-7, 64.15) -> (-7, -7)
  line L30 (-7, -7) -> (254.65, -7)
  line L31 (254.65, -7) -> (254.65, 64.15)
  line L32 (-1, -1) -> (-6, -1)
  line L33 (-6, -1) -> (-6, 5)
  line L34 (-6, 5) -> (-1, 5)
  line L35 (-1, 5) -> (-1, -1)
  line L36 (-1, 58.15) -> (-6, 58.15)
  line L37 (-6, 58.15) -> (-6, 52.15)
  line L38 (-6, 52.15) -> (-1, 52.15)
  line L39 (-1, 52.15) -> (-1, 58.15)
  line L40 (248.65, -1) -> (253.65, -1)
  line L41 (253.65, -1) -> (253.65, 5)
  line L42 (253.65, 5) -> (248.65, 5)
  line L43 (248.65, 5) -> (248.65, -1)
  line L44 (248.65, 58.15) -> (253.65, 58.15)
  line L45 (253.65, 58.15) -> (253.65, 52.15)
  line L46 (253.65, 52.15) -> (248.65, 52.15)
  line L47 (248.65, 52.15) -> (248.65, 58.15)
  dimension "d21" = 5
  dimension "d22" = 6
  dimension "d23" = 5
  dimension "d24" = 6
  dimension "d25" = 5
  dimension "d26" = 6
  dimension "d27" = 5
  dimension "d28" = 6
  constraint horizontal L32
  constraint vertical L33
  constraint horizontal L34
  constraint vertical L35
  constraint coincident L7.end L8.start
  constraint horizontal L36
  constraint vertical L37
  constraint horizontal L38
  constraint vertical L39
  constraint coincident L16.end L17.start
  constraint horizontal L40
  constraint vertical L41
  constraint horizontal L42
  constraint vertical L43
  constraint coincident L6.end L7.start
  constraint horizontal L44
  constraint vertical L45
  constraint horizontal L46
  constraint vertical L47
  constraint coincident L21.end L22.start
  measures "d21" distance of L7.end L32.end
  measures "d22" distance of L7.end L34.end
  measures "d23" distance of L16.end L36.end
  measures "d24" distance of L16.end L38.end
  measures "d25" distance of L6.end L40.end
  measures "d26" distance of L6.end L42.end
  measures "d27" distance of L21.end L44.end
  measures "d28" distance of L21.end L46.end
extrude "Extrude4" cut sketch "Sketch3" against normal blind 12 contours L0 L1 L2 L22 L23 L44 L45 L46 L47 | L2 L3 L4 L5 L6 L40 L41 L42 L43 | L12 L13 L14 L15 L16 L36 L37 L38 L39 | L8 L9 L10 L11 L12 L32 L33 L34 L35 bodies 2 in component "threeu"
combine "Combine1" operation add target body 1 tool bodies 2 in component "threeu"
draft "Draft1" angle 4.3 neutral plane through (97.113, -73.675, 0) pull (0, -1, 0) 1 faces at (80.55, 5, -12) on bodies 1 in component "threeu"
fillet "Fillet1" radius 76 4 edges at (150.537, -64.15, -2.4581) (141.012, -73.675, -2.1) (97.113, -73.675, -2.1) (87.588, -64.15, -2.4581) on bodies 1 in component "threeu"
sketch "Sketch4" plane through (0, 0, 7.8) normal (0, 0, 1) x (-1, 0, 0) in component "threeu"
  line L0 (-147.6375, 57.15) -> (-147.6375, 38.1)
  line L1 (-147.6375, 38.1) -> (-90.4875, 38.1)
  line L2 (-90.4875, 38.1) -> (-90.4875, 57.15)
  line L3 (-90.4875, 57.15) -> (-14.2875, 57.15)
  line L4 (-14.2875, 57.15) -> (-14.2875, 38.1)
  line L5 (-14.2875, 38.1) -> (0, 38.1)
  line L6 (0, 38.1) -> (0, 0)
  line L7 (0, 0) -> (-247.65, 0)
  line L8 (-247.65, 0) -> (-247.65, 38.1)
  line L9 (-247.65, 38.1) -> (-242.8875, 38.1)
  line L10 (-242.8875, 38.1) -> (-242.8875, 57.15)
  line L11 (-242.8875, 57.15) -> (-147.6375, 57.15)
  line L12 (-100.0125, 47.625) -> (-138.1125, 47.625)
  line L13 (-138.1125, 47.625) -> (-138.1125, 66.675)
  line L14 (-138.1125, 66.675) -> (-100.0125, 66.675)
  line L15 (-100.0125, 66.675) -> (-100.0125, 47.625)
  arc A0 (-86.755, 68.9125) -> (-113.2356, 73.675) centre (-113.2356, -2.325) ccw
  line L16 (-113.2356, 73.675) -> (-124.8894, 73.675)
  arc A1 (-124.8894, 73.675) -> (-151.37, 68.9125) centre (-124.8894, -2.325) ccw
  arc A2 (-177.8505, 64.15) -> (-151.37, 68.9125) centre (-177.8505, 140.15) ccw
  line L17 (-177.8505, 64.15) -> (-254.65, 64.15)
  line L18 (-254.65, 64.15) -> (-254.65, -7)
  line L19 (-254.65, -7) -> (7, -7)
  line L20 (7, -7) -> (7, 64.15)
  line L21 (7, 64.15) -> (-60.2745, 64.15)
  arc A3 (-86.755, 68.9125) -> (-60.2745, 64.15) centre (-60.2745, 140.15) ccw
  line L22 (0.3, 38.4) -> (0.3, -0.3)
  line L23 (0.3, -0.3) -> (-247.95, -0.3)
  line L24 (-247.95, -0.3) -> (-247.95, 38.4)
  line L25 (-247.95, 38.4) -> (-243.1875, 38.4)
  line L26 (-243.1875, 38.4) -> (-243.1875, 57.45)
  line L27 (-243.1875, 57.45) -> (-147.3375, 57.45)
  line L28 (-147.3375, 57.45) -> (-147.3375, 38.4)
  line L29 (-147.3375, 38.4) -> (-90.7875, 38.4)
  line L30 (-90.7875, 38.4) -> (-90.7875, 57.45)
  line L31 (-90.7875, 57.45) -> (-13.9875, 57.45)
  line L32 (-13.9875, 57.45) -> (-13.9875, 38.4)
  line L33 (-13.9875, 38.4) -> (0.3, 38.4)
  line L34 (-138.4125, 66.975) -> (-99.7125, 66.975)
  line L35 (-99.7125, 66.975) -> (-99.7125, 47.325)
  line L36 (-99.7125, 47.325) -> (-138.4125, 47.325)
  line L37 (-138.4125, 47.325) -> (-138.4125, 66.975)
  dimension "d35" = -0.3
  dimension "d36" = -0.3
extrude "Extrude5" cut sketch "Sketch4" against normal blind 7.8 contours L22 L23 L24 L25 L26 L27 L28 L29 L30 L31 L32 L33 | L34 L35 L36 L37 bodies 1 in component "threeu"
delete_body "RemoveBody1" bodies 2 in component "threeu"
extrude "Extrude6" add sketch "plate-2023-07-07T18_42_50.088Z" against normal blind 1.5 separate body contours L130 L161 L162 L163 L164 | L162 L163 L164 L168 L172 L175 L179 L180 | L133 L147 L151 L152 L153 L156 L157 L160 L167 L168 L171 L172 L175 L176 L177 L178 L219 L229 | L153 L177 L206 L207 L215 L216 L249 L250 | L157 L160 L201 L202 L213 L214 L253 L254 | L206 L207 L215 L216 L247 L249 L250 | L201 L202 L213 L214 L239 L253 L254 | L216 L243 L247 L248 L252 | L214 L235 L236 L239 L256 | L147 L205 L229 L230 L232 | L242 L243 L244 L245 L246 A151 L248 L252 | L151 L203 L217 L218 L219 | L235 A150 L236 L237 L238 L240 L241 L256 | L205 L228 L230 L231 L232 A149 L233 L234 | L203 L217 L218 L220 L221 L222 L223 A148 makes body 3 in component "threeu"
fillet "Fillet2" radius 3 16 edges at (253.65, -52.15, -6.8092) (253.65, -58.15, -6.5837) (248.65, -52.15, -6.8092) (248.65, -5, -8.5818) (253.65, -5, -8.5818) (253.65, 1, -8.8074) (-1, -52.15, -6.8092) (-6, -52.15, -6.8092) (-6, -58.15, -6.5837) (-6, 1, -8.8074) (-6, -5, -8.5818) (-1, -5, -8.5818) (247.65, -4, -0.75) (247.65, -53.15, -0.75) (0, -53.15, -0.75) (0, -4, -0.75) on bodies 1 3 in component "threeu"
fillet "Fillet3" radius 1 8 edges at (-5, -57.15, -0.75) (-5, -53.15, -0.75) (-5, -4, -0.75) (-5, 0, -0.75) (252.65, 0, -0.75) (252.65, -4, -0.75) (252.65, -53.15, -0.75) (252.65, -57.15, -0.75) on bodies 3 in component "threeu"
fillet "Fillet4" radius 8 8 edges at (148.0517, -58.15, -6.5837) (138.5267, -67.675, -6.2256) (90.0733, -58.15, -6.5837) (99.5983, -67.675, -6.2256) (147.6375, -57.15, -0.75) (138.1125, -66.675, -0.75) (90.4875, -57.15, -0.75) (100.0125, -66.675, -0.75) on bodies 1 3 in component "threeu"
fillet "Fillet5" radius 1.5 16 edges at (243.1875, -38.4, 3.9) (247.95, -38.4, 3.9) (247.95, 0.3, 3.9) (243.1875, -57.45, 3.9) (138.4125, -66.975, 3.9) (138.4125, -47.325, 3.9) (147.3375, -57.45, 3.9) (147.3375, -38.4, 3.9) (99.7125, -66.975, 3.9) (99.7125, -47.325, 3.9) (90.7875, -57.45, 3.9) (90.7875, -38.4, 3.9) (13.9875, -57.45, 3.9) (13.9875, -38.4, 3.9) (-0.3, -38.4, 3.9) (-0.3, 0.3, 3.9) on bodies 1 in component "threeu"
fillet "Fillet6" radius 5 4 edges at (-7, -64.15, -2.4581) (-7, 7, -5.133) (254.65, -64.15, -2.4581) (254.65, 7, -5.133) on bodies 1 in component "threeu"
chamfer "Chamfer1" distance 0.5 angle 45 46 edges at (-5.5355, -62.6855, -12.8263) (29.1373, -64.15, -12.7162) (73.7272, -65.3501, -12.626) (99.7829, -72.4749, -12.0902) (119.0625, -73.675, -12) (138.3421, -72.4749, -12.0902) (164.3978, -65.3501, -12.626) (213.7502, -64.15, -12.7162) (253.1855, -62.6855, -12.8263) (254.65, -28.575, -15.3911) (253.1855, 5.5355, -17.9559) (123.825, 7, -18.066) (-5.5355, 5.5355, -17.9559) (-7, -28.575, -15.3911) (99.7125, -57.15, 7.8) (100.1518, -47.7643, 7.8) (119.0625, -47.325, 7.8) (137.9732, -47.7643, 7.8) (138.4125, -57.15, 7.8) (137.9732, -66.5357, 7.8) (119.0625, -66.975, 7.8) (100.1518, -66.5357, 7.8) (90.7875, -47.925, 7.8) (90.3482, -57.0107, 7.8) (52.3875, -57.45, 7.8) (14.4268, -57.0107, 7.8) (13.9875, -47.925, 7.8) (13.5482, -38.8393, 7.8) (6.8437, -38.4, 7.8) (0.1393, -37.9607, 7.8) (-0.3, -19.05, 7.8) (0.1393, -0.1393, 7.8) (123.825, 0.3, 7.8) (247.5107, -0.1393, 7.8) (247.95, -19.05, 7.8) (247.5107, -37.9607, 7.8) (245.5688, -38.4, 7.8) (243.6268, -38.8393, 7.8) (243.1875, -47.925, 7.8) (242.7482, -57.0107, 7.8) (195.2625, -57.45, 7.8) (147.7768, -57.0107, 7.8) (147.3375, -47.925, 7.8) (146.8982, -38.8393, 7.8) (119.0625, -38.4, 7.8) (91.2268, -38.8393, 7.8) on bodies 1 in component "threeu"
fillet "Fillet7" radius 1 14 edges at (73.7272, -65.3501, 7.8) (99.7829, -72.4749, 7.8) (119.0625, -73.675, 7.8) (138.3421, -72.4749, 7.8) (164.3978, -65.3501, 7.8) (213.7502, -64.15, 7.8) (253.1855, -62.6855, 7.8) (254.65, -28.575, 7.8) (253.1855, 5.5355, 7.8) (123.825, 7, 7.8) (-5.5355, 5.5355, 7.8) (-7, -28.575, 7.8) (-5.5355, -62.6855, 7.8) (29.1373, -64.15, 7.8) on bodies 1 in component "threeu"
component "threeu" placed x (1, 0, 0) y (0, 1, 0) z (0, 0, 1) at (0, 0, 0)
equation "d5 = ( 19.05 * 2 ) * 1 mm"
